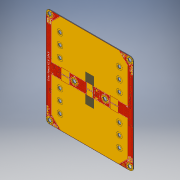
# Autodesk Inventor part: SolarPanel_PCB
Saved by Autodesk Inventor 2018 (Build 220112000, 112)
## iProperties
Created: 2018-11-29
Part Number: SolarPanel_PCB
Material: Epoxy Resin
Document SubType Name: Modeling
Designer: Bradley
Density: 1.14 g/cm^3
Appearance: Smooth - Dark Gray
Author: Bradley
Autodesk Inventor part; units mm, degrees
ref_plane "YZ Plane" through (0, 0, 0) normal (1, 0, 0) x (0, 1, 0)
ref_plane "XZ Plane" through (0, 0, 0) normal (0, 1, 0) x (-1, 0, 0)
ref_plane "XY Plane" through (0, 0, 0) normal (0, 0, 1) x (1, 0, 0)
sketch "Sketch1" plane through (0, 0, 0) normal (0, 1, 0) x (-1, 0, 0)
  line L0 (36.5, -45) -> (-36.5, -45)
  line L1 (-39.5, -42) -> (-39.5, 42)
  line L2 (-36.5, 45) -> (36.5, 45)
  line L3 (39.5, 42) -> (39.5, -42)
  line L4 (39.5, -45) -> (-39.5, 45) construction
  line L5 (-39.5, -45) -> (39.5, 45) construction
  arc A0 (39.5, 42) -> (36.5, 45) centre (36.5, 42) ccw
  arc A1 (36.5, -45) -> (39.5, -42) centre (36.5, -42) ccw
  arc A2 (-39.5, -42) -> (-36.5, -45) centre (-36.5, -42) ccw
  arc A3 (-36.5, 45) -> (-39.5, 42) centre (-36.5, 42) ccw
  circle A4 centre (36.5, 42) radius 1.65
  circle A5 centre (-36.5, 42) radius 1.65
  circle A6 centre (-36.5, -42) radius 1.65
  circle A7 centre (36.5, -42) radius 1.65
  line L6 (14, 0) -> (-14, 0) construction
  circle A8 centre (14, 0) radius 1.65
  circle A9 centre (-14, 0) radius 1.65
  point P0 (0, 0)
  point P1 (0, 0)
  dimension "d0" = 79
  dimension "d1" = 90
  dimension "d2" = 3
  dimension "d3" = 3.3
  dimension "d4" = 28
  constraints: 14 end point, 10 centre point, 8 equal radius, 8 point on circle, 8 point on line, 8 tangent, 6 coincident, 4 midpoint, 2 horizontal, 2 parallel, 1 perpendicular
  measures "d0" distance of L4.end L5.end
  measures "d1" distance of L5.end L4.start
  measures "d2" radius of A0
  measures "d3" diameter of A4
  measures "d4" distance of L6.start L6.end
extrude "Extrusion1" add sketch "Sketch1" along normal mid plane 0.6
sketch "Sketch2" plane through (0, -0.3, 0) normal (0, -1, 0) x (1, 0, 0)
  circle A0 centre (14, 0) radius 1.65 projected
  circle A1 centre (-14, 0) radius 1.65 projected
  circle A2 centre (-36.5, -42) radius 1.65 projected
  circle A3 centre (36.5, -42) radius 1.65 projected
  circle A4 centre (36.5, 42) radius 1.65 projected
  circle A5 centre (-36.5, 42) radius 1.65 projected
  line L0 (-39.5, 42) -> (-39.5, -42) projected
  arc A6 (-39.5, -42) -> (-36.5, -45) centre (-36.5, -42) ccw projected
  line L1 (-36.5, -45) -> (36.5, -45) projected
  arc A7 (36.5, -45) -> (39.5, -42) centre (36.5, -42) ccw projected
  line L2 (39.5, -42) -> (39.5, 42) projected
  arc A8 (39.5, 42) -> (36.5, 45) centre (36.5, 42) ccw projected
  line L3 (36.5, 45) -> (-36.5, 45) projected
  arc A9 (-36.5, 45) -> (-39.5, 42) centre (-36.5, 42) ccw projected
  line L4 (-39.5, 42) -> (-39.5, -42) projected
  line L5 (39.5, -42) -> (39.5, 42) projected
  line L6 (-39.5, 44.9957) -> (39.5, 44.9957) construction
  line L7 (39.5, 44.9957) -> (39.5, -44.9957) construction
  line L8 (39.5, -44.9957) -> (-39.5, -44.9957) construction
  line L9 (-39.5, -44.9957) -> (-39.5, 44.9957) construction
  point P0 (0, 0)
  point P1 (39.5, 0)
  point P2 (39.5, 0)
  point P3 (39.5, 0)
  constraints: 4 midpoint, 2 collinear, 2 other
decal "Decal1"
sketch "Sketch3" plane through (0, 0.3, 0) normal (0, 1, 0) x (1, 0, 0)
  circle A0 centre (14, 0) radius 1.65 projected
  circle A1 centre (-14, 0) radius 1.65 projected
  circle A2 centre (-36.5, 42) radius 1.65 projected
  circle A3 centre (36.5, 42) radius 1.65 projected
  circle A4 centre (36.5, -42) radius 1.65 projected
  circle A5 centre (-36.5, -42) radius 1.65 projected
  line L0 (-39.5, 42) -> (-39.5, -42) projected
  arc A6 (-39.5, -42) -> (-36.5, -45) centre (-36.5, -42) ccw projected
  line L1 (-36.5, -45) -> (36.5, -45) projected
  arc A7 (36.5, -45) -> (39.5, -42) centre (36.5, -42) ccw projected
  line L2 (39.5, -42) -> (39.5, 42) projected
  arc A8 (39.5, 42) -> (36.5, 45) centre (36.5, 42) ccw projected
  line L3 (36.5, 45) -> (-36.5, 45) projected
  arc A9 (-36.5, 45) -> (-39.5, 42) centre (-36.5, 42) ccw projected
  line L4 (39.5, -42) -> (39.5, 42) projected
  line L5 (39.5, -44.9957) -> (-39.5, -44.9957) construction
  line L6 (-39.5, -44.9957) -> (-39.5, 44.9957) construction
  line L7 (-39.5, 44.9957) -> (39.5, 44.9957) construction
  line L8 (39.5, 44.9957) -> (39.5, -44.9957) construction
  point P0 (0, 0)
  point P1 (39.5, 0)
  point P2 (39.5, 0)
  point P3 (39.5, 0)
  constraints: 4 midpoint, 2 collinear, 2 other
decal "Decal2"
sketch "Sketch4" plane through (0, -0.3, 0) normal (0, -1, 0) x (1, 0, 0)
  point P0 (0, 0)
  point P1 (27, -22)
  point P2 (27, 32)
  point P3 (27, 22)
  point P4 (27, 12)
  point P5 (-27, 32)
  point P6 (27, -12)
  point P7 (-27, 22)
  point P8 (-27, 12)
  point P9 (-27, -32)
  point P10 (-27, -22)
  point P11 (27, -32)
  point P12 (-27, -12)
  constraints: 12 other
hole "Hole1" at (27, -0.3, -22) at (27, -0.3, 32) at (27, -0.3, 22) at (27, -0.3, 12) at (-27, -0.3, 32) at (27, -0.3, -12) at (-27, -0.3, 22) at (-27, -0.3, 12) at (-27, -0.3, -32) at (-27, -0.3, -22) at (27, -0.3, -32) at (-27, -0.3, -12) direction (0, 1, 0) diameter 3 end through all
sketch "Sketch5" plane through (0, -0.3, 0) normal (0, -1, 0) x (1, 0, 0)
  point P0 (0, 0)
  point P1 (-12.374, -1.626)
  point P2 (-15.626, -1.626)
  point P3 (-14, -2.3)
  point P4 (-15.626, 1.626)
  point P5 (-14, 2.3)
  point P6 (-12.374, 1.626)
  point P7 (-11.7, 0)
  point P8 (-16.3, 0)
  point P9 (34.874, -40.374)
  point P10 (38.126, -43.626)
  point P11 (34.874, -43.626)
  point P12 (36.5, -39.7)
  point P13 (38.126, -40.374)
  point P14 (38.8, -42)
  point P15 (34.2, -42)
  point P16 (36.5, -44.3)
  point P17 (34.874, 40.374)
  point P18 (36.5, 39.7)
  point P19 (34.874, 43.626)
  point P20 (36.5, 44.3)
  point P21 (38.126, 43.626)
  point P22 (38.8, 42)
  point P23 (34.2, 42)
  point P24 (38.126, 40.374)
  point P25 (-34.874, 40.374)
  point P26 (-38.126, 40.374)
  point P27 (-36.5, 39.7)
  point P28 (-38.126, 43.626)
  point P29 (-36.5, 44.3)
  point P30 (-34.874, 43.626)
  point P31 (-34.2, 42)
  point P32 (15.626, -1.626)
  point P33 (12.374, -1.626)
  point P34 (-34.874, -43.626)
  point P35 (14, -2.3)
  point P36 (12.374, 1.626)
  point P37 (14, 2.3)
  point P38 (15.626, 1.626)
  point P39 (-38.126, -43.626)
  point P40 (-38.8, 42)
  point P41 (-38.126, -40.374)
  point P42 (-36.5, -39.7)
  point P43 (-34.874, -40.374)
  point P44 (-34.2, -42)
  point P45 (-38.8, -42)
  point P46 (16.3, 0)
  point P47 (11.7, 0)
  point P48 (-36.5, -44.3)
  constraints: 48 other
hole "Hole2" at (-12.374, -0.3, -1.626) at (-15.626, -0.3, -1.626) at (-14, -0.3, -2.3) at (-15.626, -0.3, 1.626) at (-14, -0.3, 2.3) at (-12.374, -0.3, 1.626) at (-11.7, -0.3, 0) at (-16.3, -0.3, 0) at (34.874, -0.3, -40.374) at (38.126, -0.3, -43.626) at (34.874, -0.3, -43.626) at (36.5, -0.3, -39.7) at (38.126, -0.3, -40.374) at (38.8, -0.3, -42) at (34.2, -0.3, -42) at (36.5, -0.3, -44.3) at (34.874, -0.3, 40.374) at (36.5, -0.3, 39.7) at (34.874, -0.3, 43.626) at (36.5, -0.3, 44.3) at (38.126, -0.3, 43.626) at (38.8, -0.3, 42) at (34.2, -0.3, 42) at (38.126, -0.3, 40.374) at (-34.874, -0.3, 40.374) at (-38.126, -0.3, 40.374) at (-36.5, -0.3, 39.7) at (-38.126, -0.3, 43.626) at (-36.5, -0.3, 44.3) at (-34.874, -0.3, 43.626) at (-34.2, -0.3, 42) at (15.626, -0.3, -1.626) at (12.374, -0.3, -1.626) at (-34.874, -0.3, -43.626) at (14, -0.3, -2.3) at (12.374, -0.3, 1.626) at (14, -0.3, 2.3) at (15.626, -0.3, 1.626) at (-38.126, -0.3, -43.626) at (-38.8, -0.3, 42) at (-38.126, -0.3, -40.374) at (-36.5, -0.3, -39.7) at (-34.874, -0.3, -40.374) at (-34.2, -0.3, -42) at (-38.8, -0.3, -42) at (16.3, -0.3, 0) at (11.7, -0.3, 0) at (-36.5, -0.3, -44.3) direction (0, 1, 0) diameter 0.45 end through all
sketch "Sketch6" plane through (0, -0.3, 0) normal (0, -1, 0) x (1, 0, 0)
  point P0 (0, 0)
  point P1 (-27.75, 0.945)
  point P2 (-36.695, -36.5)
  point P3 (-37.417, -34.833)
  point P4 (11.75, 3.5)
  point P5 (18.25, 3.5)
  point P6 (36.039, 5.211)
  point P7 (36.039, -3.228)
  point P8 (37.252, -10.392)
  point P9 (37, 13.888)
  point P10 (35.047, 38.56)
  point P11 (-29.25, -44.04)
  point P12 (26.235, 1.5)
  point P13 (2.985, 2.5)
  point P14 (6.035, -1.035)
  point P15 (6.035, 0.535)
  point P16 (4.465, -1.25)
  point P17 (31, 41)
  point P18 (-33.25, -44.4)
  point P19 (-34.44, 3.458)
  point P20 (38.39, 29.572)
  point P21 (8.75, 4.5)
  point P22 (2.985, 3.44)
  point P23 (-36.12, -16.831)
  point P24 (-36.396, -18.646)
  point P25 (35, 33.69)
  point P26 (35, 5)
  point P27 (10, -4)
  point P28 (4.465, -2.06)
  point P29 (-23.01, 0)
  point P30 (23.01, 0)
  point P31 (-31.656, 2.294)
  point P32 (-36.638, 33.75)
  point P33 (-36.145, -3.022)
  point P34 (8.708, -2.792)
  point P35 (8.01, 2.75)
  point P36 (35.479, 3.859)
  point P37 (37, 21.419)
  point P38 (37.454, 17.611)
  point P39 (37.5, -8.585)
  point P40 (38.875, -9.597)
  point P41 (37.113, 15.25)
  point P42 (-28.25, -43.68)
  point P43 (-32.26, -41.189)
  point P44 (-35.5, -37.46)
  point P45 (37.165, 6.415)
  point P46 (37.165, 3.962)
  point P47 (0, 0)
  point P48 (13.555, -4.25)
  point P49 (18.25, -4.25)
  point P50 (26, -1.5)
  point P51 (-32.306, 2.944)
  point P52 (36.38, 9.38)
  point P53 (7.25, -0.25)
  point P54 (-35.75, 33.75)
  point P55 (-36.5, -19.791)
  point P56 (4.465, 1.635)
  point P57 (-26.395, 0.63)
  point P58 (-27.79, -4)
  point P59 (-26.245, -4)
  point P60 (-30, -3.915)
  point P61 (-34.44, 4.25)
  point P62 (-29.321, -3.448)
  point P63 (-35.313, -17.51)
  point P64 (-35.223, 8.473)
  point P65 (-35, -16.75)
  point P66 (-35, 7.5)
  point P67 (2.985, 4.25)
  point P68 (6.035, 4.523)
  point P69 (35.039, 35.789)
  point P70 (35.945, 8.67)
  point P71 (35.585, 7.5)
  point P72 (35, 35)
  point P73 (-35.595, -19.845)
  point P74 (-32.5, -42.79)
  point P75 (35.81, -5.889)
  point P76 (35.81, -10)
  point P77 (36.64, 10.536)
  point P78 (36.64, 11.706)
  point P79 (-31.5, -40.92)
  point P80 (-29.75, -42.54)
  point P81 (-3.015, -2.188)
  point P82 (-27.595, 2.345)
  point P83 (-10.155, -2.25)
  point P84 (-11.534, -2.466)
  point P85 (-33.855, -2.895)
  point P86 (-34.415, -0.5)
  point P87 (36.64, 14.648)
  point P88 (36.64, 12.516)
  point P89 (-34.44, -37.4)
  point P90 (37.789, 31)
  point P91 (3, -0.785)
  point P92 (3, -4)
  point P93 (-26.235, -1.75)
  point P94 (-36.145, -5.186)
  point P95 (-28.544, 4.544)
  point P96 (-8.985, 3.75)
  point P97 (-18.25, 0.75)
  point P98 (37.085, 32.75)
  point P99 (-34.415, 1.25)
  point P100 (-32.466, 0.657)
  point P101 (36.879, 28.446)
  point P102 (-26.235, -0.94)
  point P103 (-28.565, -0.585)
  constraints: 101 other
hole "Hole3" at (-27.75, -0.3, 0.945) at (-36.695, -0.3, -36.5) at (-37.417, -0.3, -34.833) at (11.75, -0.3, 3.5) at (18.25, -0.3, 3.5) at (36.039, -0.3, 5.211) at (36.039, -0.3, -3.228) at (37.252, -0.3, -10.392) at (37, -0.3, 13.888) at (35.047, -0.3, 38.56) at (-29.25, -0.3, -44.04) at (26.235, -0.3, 1.5) at (2.985, -0.3, 2.5) at (6.035, -0.3, -1.035) at (6.035, -0.3, 0.535) at (4.465, -0.3, -1.25) at (31, -0.3, 41) at (-33.25, -0.3, -44.4) at (-34.44, -0.3, 3.458) at (38.39, -0.3, 29.572) at (8.75, -0.3, 4.5) at (2.985, -0.3, 3.44) at (-36.12, -0.3, -16.831) at (-36.396, -0.3, -18.646) at (35, -0.3, 33.69) at (35, -0.3, 5) at (10, -0.3, -4) at (4.465, -0.3, -2.06) at (-23.01, -0.3, 0) at (23.01, -0.3, 0) at (-31.656, -0.3, 2.294) at (-36.638, -0.3, 33.75) at (-36.145, -0.3, -3.022) at (8.708, -0.3, -2.792) at (8.01, -0.3, 2.75) at (35.479, -0.3, 3.859) at (37, -0.3, 21.419) at (37.454, -0.3, 17.611) at (37.5, -0.3, -8.585) at (38.875, -0.3, -9.597) at (37.113, -0.3, 15.25) at (-28.25, -0.3, -43.68) at (-32.26, -0.3, -41.189) at (-35.5, -0.3, -37.46) at (37.165, -0.3, 6.415) at (37.165, -0.3, 3.962) at (0, -0.3, 0) at (13.555, -0.3, -4.25) at (18.25, -0.3, -4.25) at (26, -0.3, -1.5) direction (0, 1, 0) diameter 0.3 end through all and at (-32.306, -0.3, 2.944) (36.38, -0.3, 9.38) (7.25, -0.3, -0.25) (-35.75, -0.3, 33.75) (-36.5, -0.3, -19.791) (4.465, -0.3, 1.635) (-26.395, -0.3, 0.63) (-27.79, -0.3, -4) (-26.245, -0.3, -4) (-30, -0.3, -3.915) (-34.44, -0.3, 4.25) (-29.321, -0.3, -3.448) (-35.313, -0.3, -17.51) (-35.223, -0.3, 8.473) (-35, -0.3, -16.75) (-35, -0.3, 7.5) (2.985, -0.3, 4.25) (6.035, -0.3, 4.523) (35.039, -0.3, 35.789) (35.945, -0.3, 8.67) (35.585, -0.3, 7.5) (35, -0.3, 35) (-35.595, -0.3, -19.845) (-32.5, -0.3, -42.79) (35.81, -0.3, -5.889) (35.81, -0.3, -10) (36.64, -0.3, 10.536) (36.64, -0.3, 11.706) (-31.5, -0.3, -40.92) (-29.75, -0.3, -42.54) (-3.015, -0.3, -2.188) (-27.595, -0.3, 2.345) (-10.155, -0.3, -2.25) (-11.534, -0.3, -2.466) (-33.855, -0.3, -2.895) (-34.415, -0.3, -0.5) (36.64, -0.3, 14.648) (36.64, -0.3, 12.516) (-34.44, -0.3, -37.4) (37.789, -0.3, 31) (3, -0.3, -0.785) (3, -0.3, -4) (-26.235, -0.3, -1.75) (-36.145, -0.3, -5.186) (-28.544, -0.3, 4.544) (-8.985, -0.3, 3.75) (-18.25, -0.3, 0.75) (37.085, -0.3, 32.75) (-34.415, -0.3, 1.25) (-32.466, -0.3, 0.657) (36.879, -0.3, 28.446) (-26.235, -0.3, -0.94) (-28.565, -0.3, -0.585)
body "Solid1"
